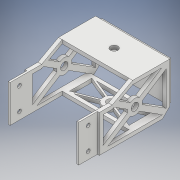
# Autodesk Inventor part: Biceps1 v2
Saved by Autodesk Inventor 2018 (Build 220112000, 112)
## iProperties
Created: 2018-04-10
Part Number: Biceps1 v2
Material: Plastique ABS
Document SubType Name: Modeling
Designer: Thomas
Density: 1.06 g/cm^3
Appearance: Lisse - Blanc
Author: Thomas
Autodesk Inventor part; units mm, degrees
ref_plane "YZ Plane" through (0, 0, 0) normal (1, 0, 0) x (0, 1, 0)
ref_plane "XZ Plane" through (0, 0, 0) normal (0, 1, 0) x (-1, 0, 0)
ref_plane "XY Plane" through (0, 0, 0) normal (0, 0, 1) x (1, 0, 0)
sketch "Esquisse1" plane through (0, 0, 0) normal (0, 0, 1) x (1, 0, 0)
  line L0 (0, 0) -> (100, 0)
  line L1 (100, 0) -> (100, -50)
  line L2 (100, -50) -> (0, -50)
  line L3 (0, -50) -> (0, 0)
  dimension "d0" = 50
  dimension "d1" = 100
  constraints: 8 end point, 2 parallel, 1 horizontal, 1 perpendicular
  measures "d0" distance of L2.end L0.start
  measures "d1" distance of L1.end L2.end
extrude "Extrusion1" add sketch "Esquisse1" along normal blind 5
sketch "Esquisse2" plane through (0, 0, 5) normal (0, 0, 1) x (1, 0, 0)
  line L0 (100, 0) -> (0, 0) construction
  line L1 (0, -50) -> (100, -50) construction
  line L2 (0, 0) -> (100, -50) construction
  line L3 (0, 0) -> (0, -50) construction
  line L4 (100, 0) -> (0, -50) construction
  circle A0 centre (50, -25) radius 5
  dimension "d4" = 10
  constraints: 4 end point, 1 centre point, 1 midpoint
  measures "d4" diameter of A0
extrude "Extrusion2" cut sketch "Esquisse2" against normal blind 5
sketch "Esquisse3" plane through (0, 0, 0) normal (0, 0, -1) x (-1, 0, 0)
  line L0 (-100, 0) -> (-95, 0)
  line L1 (-95, 0) -> (-95, -50)
  line L2 (-95, -50) -> (-100, -50)
  line L3 (-100, -50) -> (-100, 0)
  line L4 (0, 0) -> (-5, 0)
  line L5 (-5, 0) -> (-5, -50)
  line L6 (-5, -50) -> (0, -50)
  line L7 (0, -50) -> (0, 0)
  dimension "d7" = 5
  dimension "d8" = 5
  constraints: 16 end point, 4 parallel, 2 horizontal, 2 perpendicular
  measures "d7" distance of L1.end L2.end
  measures "d8" distance of L5.end L6.end
extrude "Extrusion3" add sketch "Esquisse3" along normal blind 60
chamfer "Chanfrein1" distance 10 angle 45 1 edges at (97.5, 0, -60)
chamfer "Chanfrein2" distance 10 angle 45 1 edges at (2.5, 0, -60)
sketch "Esquisse4" plane through (100, -50, 5) normal (1, 0, 0) x (0, 0, -1)
  line L0 (0, 0) -> (15, -27.5984)
  line L1 (0, 50) -> (0, 0) projected
  line L2 (0, 0) -> (15, 0)
  line L3 (0, 0) -> (65, 0) projected
  line L4 (65, 0) -> (65, -70)
  line L5 (65, -70) -> (15, -70)
  line L6 (15, -27.5984) -> (15, -70)
  point P0 (5, 50)
  dimension "d17" = 15
  dimension "d18" = 70
  constraints: 10 end point, 2 vertical
  measures "d17" distance of L0.start L2.end
  measures "d18" distance of L3.end L4.end
extrude "Extrusion4" add sketch "Esquisse4" against normal blind 5
sketch "Esquisse5" plane through (100, 0, 5) normal (1, 0, 0) x (0, 0, -1)
  line L0 (65, -120) -> (15, -120) projected
  line L1 (65, -10) -> (65, -120) projected
  line L2 (15, -120) -> (65, -120)
  line L3 (65, -120) -> (65, -95)
  line L4 (65, -95) -> (15, -95)
  line L5 (15, -95) -> (15, -120)
  point P0 (5, 0)
  dimension "d21" = 25
  constraints: 8 end point, 2 parallel, 1 horizontal, 1 perpendicular, 1 point on line
  measures "d21" distance of L4.end L0.end
extrude "Extrusion5" cut sketch "Esquisse5" against normal blind 2.5
sketch "Esquisse6" plane through (97.5, 0, 5) normal (1, 0, 0) x (0, 0, -1)
  circle A0 centre (25, -107.5) radius 2.6
  circle A1 centre (55, -107.5) radius 2.6
  line L0 (15, -120) -> (15, -95) projected
  line L1 (65, -95) -> (65, -120) projected
  line L2 (15, -95) -> (65, -95) projected
  point P0 (5, 0)
  dimension "d24" = 5.2
  dimension "d25" = 5.2
  dimension "d26" = 10
  dimension "d27" = 10
  dimension "d28" = 12.5
  dimension "d29" = 12.5
  constraints: 2 centre point
  measures "d24" diameter of A0
  measures "d25" diameter of A1
  measures "d26" distance from line of L0 A0.centre
  measures "d27" distance from line of L1 A1.centre
  measures "d28" distance from line of L2 A0.centre
  measures "d29" distance from line of L2 A1.centre
extrude "Extrusion6" cut sketch "Esquisse6" against normal blind 2.5
sketch "Esquisse8" plane through (0, 0, 5) normal (0, 1, 0) x (1, 0, 0)
  line L0 (3.5, 3.5) -> (96.5, 3.5)
  line L1 (96.5, 3.5) -> (96.5, 55)
  line L2 (96.5, 55) -> (3.5, 55)
  line L3 (3.5, 55) -> (3.5, 3.5)
  point P0 (0, 5)
  constraints: 8 end point, 2 parallel, 1 horizontal, 1 perpendicular
extrude "Extrusion8" add sketch "Esquisse8" along normal blind 5
chamfer "Chanfrein5" distance 3.5 angle 45 1 edges at (96.5, 0, -24.25)
chamfer "Chanfrein6" distance 3.5 angle 45 1 edges at (50, 0, 1.5)
chamfer "Chanfrein7" distance 3.5 angle 45 1 edges at (3.5, 0, -24.25)
sketch "Esquisse9" plane through (0, 0, -60) normal (0, 0, -1) x (-1, 0, 0)
  line L0 (-5, -50) -> (0, -50) projected
  line L1 (-95, -10) -> (-95, 0) projected
  line L2 (-5, -50) -> (-95, -50)
  line L3 (-95, -50) -> (-95, -10)
  line L4 (-95, -10) -> (-5, -10)
  line L5 (-5, -10) -> (-5, -50)
  point P0 (0, 0)
  constraints: 8 end point, 2 parallel, 1 horizontal, 1 perpendicular
extrude "Extrusion9" add sketch "Esquisse9" against normal blind 5
sketch "Esquisse10" plane through (0, -50, -60) normal (-1, 0, 0) x (0, 0, 1)
  line L0 (50, -27.5984) -> (65, 0) projected
  line L1 (65, 0) -> (50, -27.5984)
  line L2 (50, -70) -> (50, -27.5984) projected
  line L3 (50, -27.5984) -> (50, -70)
  line L4 (0, -70) -> (50, -70) projected
  line L5 (50, -70) -> (0, -70)
  line L6 (0, -70) -> (0, 0)
  line L7 (0, 0) -> (65, 0)
  point P0 (60, 50)
  constraints: 10 end point, 3 collinear, 1 horizontal
extrude "Extrusion10" add sketch "Esquisse10" against normal blind 5
sketch "Esquisse11" plane through (0, 0, -50) normal (-1, 0, 0) x (0, 0, 1)
  line L0 (40, -77.5984) -> (40, -120) projected
  line L1 (-10, -120) -> (40, -120)
  line L2 (40, -120) -> (40, -95)
  line L3 (40, -95) -> (-10, -95)
  line L4 (-10, -95) -> (-10, -120)
  point P0 (50, 0)
  dimension "d63" = 25
  constraints: 8 end point, 2 parallel, 1 horizontal, 1 perpendicular, 1 point on line
  measures "d63" distance of L3.end L1.start
extrude "Extrusion11" cut sketch "Esquisse11" against normal blind 2.5
sketch "Esquisse12" plane through (2.5, 0, -50) normal (-1, 0, 0) x (0, 0, 1)
  circle A0 centre (0, -107.5) radius 2.6 projected
  circle A1 centre (0, -107.5) radius 2.6
  circle A2 centre (30, -107.5) radius 2.6 projected
  circle A3 centre (30, -107.5) radius 2.6
  point P0 (50, 0)
  constraints: 2 centre point, 2 coincident
extrude "Extrusion12" cut sketch "Esquisse12" against normal blind 2.5
sketch "Esquisse13" plane through (100, -95, -10) normal (1, 0, 0) x (0, 0, -1)
  line L0 (-10, 90) -> (35.5969, 90)
  line L1 (-10, 47.7175) -> (-10, 90)
  line L2 (-15, 45) -> (-15, 95) projected
  line L3 (-15, 45) -> (0, 17.4016) projected
  line L4 (-10, 47.7175) -> (-10, 45)
  line L5 (-15, 45) -> (0, 17.4016) projected
  line L6 (-15, 95) -> (40, 95) projected
  line L7 (35.5969, 90) -> (40, 90)
  line L8 (45, 85) -> (45, 45) projected
  line L9 (45, 85) -> (45, 5.9149)
  line L10 (5, 17.4016) -> (5, 5)
  line L11 (5, 5) -> (45, 5)
  line L12 (45, 5) -> (45, 5.9149)
  line L13 (0, 0) -> (50, 0) projected
  line L14 (0, 17.4016) -> (0, 0) projected
  line L15 (5, 17.4016) -> (5, 17.4016)
  line L16 (5, 17.4016) -> (-10, 45)
  line L17 (40, 90) -> (45, 85)
  line L18 (45, 45) -> (45, 85) construction
  circle A0 centre (17.2708, 47.8542) radius 5
  circle A1 centre (17.2708, 47.8542) radius 10
  line L19 (19.4502, 57.6138) -> (40, 90)
  line L20 (45, 85) -> (25.2526, 53.8784)
  line L21 (3.6653, 19.8572) -> (15.2197, 38.0668)
  line L22 (9.3688, 41.7257) -> (-0.1053, 26.7947)
  line L23 (-5.8908, 90) -> (15.0684, 57.6086) construction
  line L24 (19.4729, 38.0996) -> (40.8908, 5)
  line L25 (-5.8908, 90) -> (15.0684, 57.6086)
  line L26 (25.2663, 41.8482) -> (45, 11.3507)
  line L27 (-10, 83.6477) -> (9.2748, 53.8594)
  line L28 (-10, 45) -> (-10, 95) projected
  line L29 (-10, 83.6477) -> (-10, 45)
  line L30 (-10, 45) -> (-0.1053, 26.7947)
  dimension "d71" = 5
  dimension "d72" = 5
  dimension "d73" = 5
  dimension "d74" = 5
  dimension "d78" = 5
  dimension "d79" = 10
  dimension "d83" = 5
  constraints: 44 end point, 7 point on line, 4 vertical, 2 collinear, 2 horizontal, 2 perpendicular, 1 centre point, 1 coincident, 1 parallel, 10 other
  measures "d71" distance between parallel lines of L6 L0
  measures "d72" distance between parallel lines of L13 L11
  measures "d73" distance between parallel lines of L10 L14
  measures "d74" distance of L15.end L3.end
  measures "d78" radius of A0
  measures "d79" diameter of A0
  measures "d83" distance between parallel lines of L1 L2
extrude "Extrusion13" cut sketch "Esquisse13" against normal blind 5 contours L0 L7 L19 A1 L25 | L27 A1 L22 L16 L4 L1 | L8 L9 L26 A1 L20 | A1 L24 L11 L10 L16 L21 | A0
sketch "Esquisse14" plane through (0, 0, -50) normal (-1, 0, 0) x (0, 0, 1)
  line L0 (0, -5) -> (45.8908, -5) projected
  line L1 (0, -5) -> (45.8908, -5)
  line L2 (45.8908, -5) -> (50, -5)
  line L3 (0, -5) -> (-5, -10)
  line L4 (-5, -10) -> (-5, -90)
  line L5 (50, -5) -> (50, -50)
  line L6 (35, -77.5984) -> (35, -90) projected
  line L7 (50, -50) -> (35, -77.5984)
  line L8 (35, -77.5984) -> (35, -90)
  line L9 (35, -90) -> (-5, -90)
  line L10 (35, -90) -> (-0.8908, -90) projected
  line L11 (-5, -10) -> (14.7474, -41.1216) projected
  line L12 (-5, -10) -> (14.7474, -41.1216)
  line L13 (24.7803, -56.9332) -> (36.3347, -75.1428) projected
  line L14 (24.7803, -56.9332) -> (36.3347, -75.1428)
  line L15 (30.6312, -53.2743) -> (40.1053, -68.2053) projected
  line L16 (30.6312, -53.2743) -> (40.1053, -68.2053)
  arc A0 (30.6312, -53.2743) -> (30.7252, -41.1406) centre (22.7292, -47.1458) ccw projected
  line L17 (50, -11.3523) -> (30.7252, -41.1406)
  line L18 (-5, -83.6493) -> (14.7337, -53.1518) projected
  line L19 (14.7337, -53.1518) -> (-5, -83.6493)
  arc A1 (20.5271, -56.9004) -> (24.7803, -56.9332) centre (22.7292, -47.1458) ccw projected
  line L20 (-0.8908, -90) -> (20.5271, -56.9004) projected
  line L21 (-0.8908, -90) -> (20.5271, -56.9004)
  line L22 (20.5498, -37.3862) -> (0, -5) projected
  line L23 (0, -5) -> (20.5741, -37.4244)
  line L24 (24.9316, -37.3914) -> (45.8908, -5) projected
  line L25 (45.8908, -5) -> (24.9316, -37.3914)
  line L26 (-0.8908, -90) -> (35, -90)
  line L27 (35, -77.5984) -> (36.3347, -75.1428)
  line L28 (-5, -50) -> (-5, -10) projected
  line L29 (-5, -10) -> (14.7474, -41.1216)
  line L30 (-5, -10) -> (-5, -83.6493)
  arc A2 (14.7474, -41.1216) -> (14.7337, -53.1518) centre (22.7292, -47.1458) ccw projected
  line L31 (-5, -83.6493) -> (14.7337, -53.1518)
  line L32 (0, -5) -> (20.5741, -37.4244)
  line L33 (0, -5) -> (45.8908, -5)
  arc A3 (24.9316, -37.3914) -> (20.5498, -37.3862) centre (22.7292, -47.1458) ccw projected
  line L34 (24.9316, -37.3914) -> (45.8908, -5)
  line L35 (40.1053, -68.2053) -> (30.6312, -53.2743)
  line L36 (50, -50) -> (40.1053, -68.2053) projected
  line L37 (40.1053, -68.2053) -> (50, -50)
  line L38 (30.7252, -41.1406) -> (50, -11.3523) projected
  line L39 (50, -50) -> (50, -11.3523)
  line L40 (50, -11.3523) -> (30.7252, -41.1406)
  circle A4 centre (22.7292, -47.1458) radius 5
  constraints: 56 end point, 18 collinear, 2 horizontal, 1 centre point, 1 coincident, 1 perpendicular, 1 vertical
extrude "Extrusion14" cut sketch "Esquisse14" against normal blind 5 contours L0 L24 A3 L22 | L11 A2 L18 L4 | L5 L7 L15 A0 L17 | L20 A1 L13 L7 L6 L9 | A4
sketch "Esquisse15" plane through (0, 0, -60) normal (0, 0, -1) x (-1, 0, 0)
  line L0 (-5, -50) -> (-95, -50) construction
  circle A0 centre (-50, -30) radius 5
  circle A1 centre (-50, -30) radius 10
  line L1 (-95, -10) -> (-5, -10) construction
  line L2 (-95, -10) -> (-95, -50) construction
  line L3 (-5, -9.9768) -> (-5, -50) construction
  line L4 (-90, -18.6348) -> (-90, -45)
  line L5 (-90, -45) -> (-10, -45)
  line L6 (-10, -45) -> (-10, -15)
  line L7 (-10, -15) -> (-90, -15)
  line L8 (-90, -15) -> (-90, -18.6348)
  line L9 (-90, -15) -> (-59.6422, -27.3489)
  line L10 (-83.75, -15) -> (-58.7548, -25.1675)
  line L11 (-41.2507, -25.1575) -> (-16.2956, -15)
  line L12 (-10, -15) -> (-40.3559, -27.3558)
  line L13 (-10, -45) -> (-40.3578, -32.6511)
  line L14 (-16.25, -45) -> (-41.2452, -34.8325)
  line L15 (-83.7044, -45) -> (-58.7493, -34.8425)
  line L16 (-90, -45) -> (-59.6441, -32.6442)
  point P0 (0, 0)
  dimension "d90" = 20
  dimension "d89" = 10
  dimension "d91" = 5
  dimension "d92" = 5
  dimension "d93" = 5
  dimension "d94" = 5
  constraints: 30 end point, 5 perpendicular, 5 point on line, 1 centre point, 1 coincident, 1 vertical, 10 other
  measures "d89" diameter of A0
  measures "d91" distance between parallel lines of L2 L4
  measures "d92" distance between parallel lines of L1 L7
  measures "d93" distance between parallel lines of L3 L6
  measures "d94" distance between parallel lines of L0 L5
extrude "Extrusion15" cut sketch "Esquisse15" against normal blind 5 contours A0 | A1 L12 L6 L13 | A1 L10 L7 L11 | L14 L5 L15 A1 | A1 L16 L4 L8 L9
